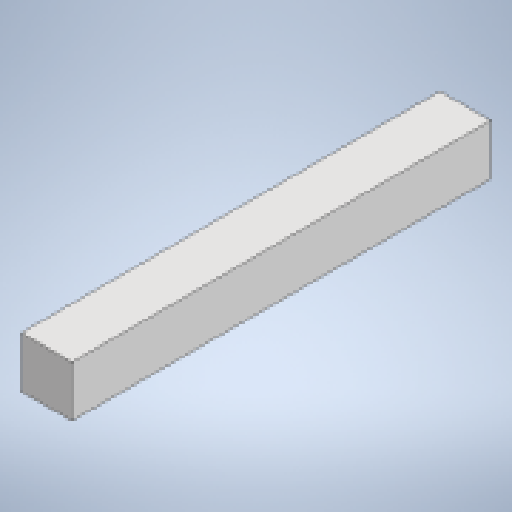
# Autodesk Inventor part: Refuerzo superior
Saved by Autodesk Inventor 2024 (Build 280153000, 153)
## iProperties
Created: 2025-03-01
Part Number: Refuerzo superior
Material: Genérico
Document SubType Name: Modeling
Designer: sergi
Density: 1 g/cm^3
Appearance: Valor por defecto
Author: sergi
Autodesk Inventor part; units mm, degrees
ref_plane "YZ Plane" through (0, 0, 0) normal (1, 0, 0) x (0, 1, 0)
ref_plane "XZ Plane" through (0, 0, 0) normal (0, 1, 0) x (-1, 0, 0)
ref_plane "XY Plane" through (0, 0, 0) normal (0, 0, 1) x (1, 0, 0)
sketch "Boceto1" plane through (0, 0, 0) normal (0, 1, 0) x (-1, 0, 0)
  line L0 (0, 0) -> (8, 0)
  line L1 (8, 0) -> (8, 66)
  line L2 (8, 66) -> (0, 66)
  line L3 (0, 66) -> (0, 0)
  dimension "d0" = 8
  dimension "d1" = 66
  constraints: 8 end point, 2 parallel, 1 horizontal, 1 perpendicular
  measures "d0" distance of L2.end L1.end
  measures "d1" distance of L1.end L0.end
extrude "Extrusión1" add sketch "Boceto1" along normal blind 8
ref_plane "Plano de trabajo1" through (-12.4, -21.9, 10) normal (0, 0, 1) x (1, 0, 0)
sketch "Boceto2" plane through (-12.4, -21.9, 10) normal (0, 0, 1) x (1, 0, 0)
  line L0 (4.4, 21.9) -> (12.4, 21.9) projected
  line L1 (12.4, 21.9) -> (12.4, 29.9) projected
  line L2 (4.4, 29.9) -> (12.4, 29.9) projected
  line L3 (4.4, 21.9) -> (4.4, 29.9) projected
  line L4 (12.5, -18.18) -> (4.3, -18.18) projected
  line L5 (4.3, -18.18) -> (4.3, -9.98) projected
  line L6 (4.3, -9.98) -> (12.5, -9.98) projected
  line L7 (12.5, -9.98) -> (12.5, -18.18) projected
  line L8 (4.3, 30) -> (12.5, 30) projected
  line L9 (12.5, 30) -> (12.5, 21.8) projected
  line L10 (12.5, 21.8) -> (4.3, 21.8) projected
  line L11 (4.3, 21.8) -> (4.3, 30) projected
  line L12 (17.5, 35) -> (2.5, 35) projected
  line L13 (2.5, 35) -> (-17.5, -35) projected
  line L14 (-17.5, -35) -> (17.5, -35) projected
  line L15 (17.5, -35) -> (17.5, 35) projected
  line L16 (12.5, 21.8) -> (17.5, 21.8)
  line L17 (4.3, 21.8) -> (-1.2714, 21.8)
  line L18 (4.3, 21.8) -> (14.2355, 21.8) construction
  line L19 (4.3, 21.8) -> (2.5, 35)
  line L20 (12.4, 21.9) -> (17.5, 21.9)
  line L21 (4.4, 21.9) -> (3.9852, 21.9)
  line L22 (4.4, 21.9) -> (4.8148, 21.9) construction
  point P0 (4.2864, 21.9)
  dimension "d4" = 180
  dimension "d22" = 180
  constraints: 14 end point, 3 point on line, 2 horizontal, 1 collinear, 1 perpendicular
  measures "d4" angle of L17 L18
  measures "d22" angle of L21 L22
ref_plane "Plano de trabajo2" through (-29.9, -56.9, 56) normal (0, 0, -1) x (0, 1, 0)
extrude "Extrusión2" add sketch "Boceto2" along normal up to surface (46 mm away) contours L21 L11 L8 L9 L20 L1 L2 L3 | L21 L19 L12 L15 L20 L9 L8 L11
sketch "Boceto3" plane through (-8, 0, 66) normal (0, 0, 1) x (1, 0, 0)
  line L0 (0, 0) -> (8, 0) projected
  line L1 (8, 0) -> (8, 8) projected
  line L2 (0, 8) -> (8, 8) projected
  line L3 (0, 0) -> (0, 8) projected
extrude "Extrusión3" add sketch "Boceto3" along normal blind 8
sketch "Boceto4" plane through (0, 0, 0) normal (0, 0, -1) x (-1, 0, 0)
  line L0 (0, 0) -> (8, 0) projected
  line L1 (8, 0) -> (8, 8) projected
  line L2 (0, 8) -> (8, 8) projected
  line L3 (0, 0) -> (0, 8) projected
extrude "Extrusión4" add sketch "Boceto4" along normal blind 8
sketch "Boceto5" plane through (0, 8, 0) normal (0, 1, 0) x (1, 0, 0)
  line L0 (-8, -10) -> (-8, 8) projected
  line L1 (0, -74) -> (-8, -74) projected
  line L2 (0, -56) -> (0, -74) projected
  line L3 (-8, 8) -> (0, 8) projected
  line L4 (0, 8) -> (-8, 8)
  line L5 (-8, 8) -> (-8, 0)
  line L6 (-8, 0) -> (0, 0)
  line L7 (0, 0) -> (0, 8)
  line L8 (0, -74) -> (-8, -74)
  line L9 (-8, -74) -> (-8, -66)
  line L10 (-8, -66) -> (0, -66)
  line L11 (0, -66) -> (0, -74)
  line L12 (0, 8) -> (-8, 0)
  line L13 (0, -74) -> (-8, -66)
  circle A0 centre (-4, 4) radius 2.1
  circle A1 centre (-4, -70) radius 2.1
  line L14 (-8, -10) -> (0, -10) projected
  line L15 (0, -10) -> (0, 8) projected
  line L16 (0, -56) -> (-8, -56) projected
  line L17 (-8, -56) -> (-8, -74) projected
  point P0 (0, 0)
  dimension "d11" = 4.2
  dimension "d12" = 4.2
  dimension "d13" = 8
  dimension "d14" = 8
  constraints: 20 end point, 4 parallel, 3 perpendicular, 2 centre point, 2 horizontal, 2 midpoint, 2 point on line
  measures "d11" diameter of A0
  measures "d12" diameter of A1
  measures "d13" distance between parallel lines of L3 L6
  measures "d14" distance between parallel lines of L10 L1
hole "Agujero1" at (-4, 8, -4) at (-4, 8, 70) direction (0, -1, 0) diameter 4.2 end through all
